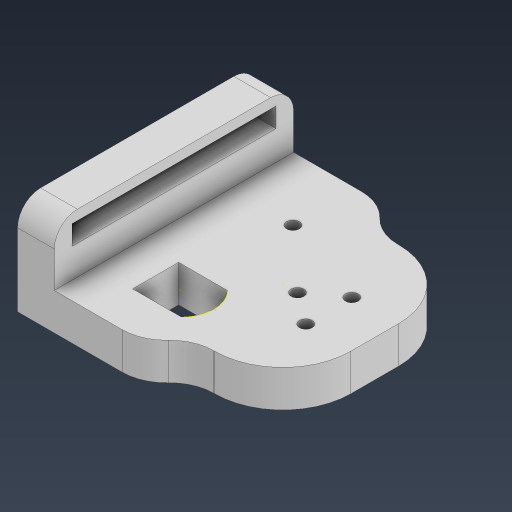
# Autodesk Inventor part: Podstawa
Saved by Autodesk Inventor 2024 (Build 280153000, 153)
## iProperties
Created: 2023-12-19
Part Number: Podstawa
Material: Generic
Document SubType Name: Modeling
Designer: Piter
Density: 1 g/cm^3
Appearance: Default
Author: Piter
Autodesk Inventor part; units mm, degrees
ref_plane "YZ Plane" through (0, 0, 0) normal (1, 0, 0) x (0, 1, 0)
ref_plane "XZ Plane" through (0, 0, 0) normal (0, 1, 0) x (-1, 0, 0)
ref_plane "XY Plane" through (0, 0, 0) normal (0, 0, 1) x (1, 0, 0)
sketch "Sketch1" plane through (0, 0, 0) normal (0, 1, 0) x (-1, 0, 0)
  line L0 (-25, 25) -> (25, 25)
  line L1 (25, 25) -> (25, -25)
  line L2 (25, -25) -> (-25, -25)
  line L3 (-25, -25) -> (-25, 25)
  line L4 (-25, 25) -> (25, -25) construction
  line L5 (25, 25) -> (-25, -25) construction
  line L6 (25, 0) -> (-25, 0)
  circle A0 centre (12.5, 15.25) radius 1.75
  line L7 (-25, 12.5) -> (0, 12.5)
  line L8 (-12.5, 12.5) -> (-12.5, 0)
  circle A1 centre (-12.5, 6.25) radius 1.75
  line L9 (25, -25) -> (-25, 25) construction
  circle A2 centre (12.5, -15.25) radius 1.75
  circle A3 centre (-12.5, -6.25) radius 1.75
  line L10 (0, 32.5) -> (50, 32.5)
  line L11 (50, 32.5) -> (50, -32.5)
  line L12 (50, -32.5) -> (0, -32.5)
  line L13 (0, -32.5) -> (0, 32.5)
  line L14 (0, 32.5) -> (50, -32.5) construction
  line L15 (50, 32.5) -> (0, -32.5) construction
  line L16 (50, -32.5) -> (29.5652, -32.5)
  line L17 (29.5652, -32.5) -> (29.5652, 32.5)
  line L18 (29.5652, 32.5) -> (50, 32.5)
  line L19 (50, 32.5) -> (50, -32.5)
  line L20 (0, 32.5205) -> (0, -32.5)
  circle A4 centre (12.5, -15.25) radius 15
  line L21 (29.5652, -32.5) -> (39.5652, -32.5)
  line L22 (39.5652, -32.5) -> (39.5652, 32.5)
  line L23 (39.5652, 32.5) -> (29.5652, 32.5)
  line L24 (29.5652, 32.5) -> (29.5652, -32.5)
  line L25 (12.5, -15.25) -> (12.5, 0)
  line L26 (-12.5, -6.25) -> (12.5, -6.25)
  circle A5 centre (-4, 0) radius 5
  circle A6 centre (-4, 0) radius 1.75
  line L27 (0, 0) -> (-4, 0)
  point P0 (0, -12.5)
  point P1 (-12.5, -12.5)
  point P2 (0, 25)
  point P3 (0, -25)
  point P4 (0, 25)
  point P5 (0, -25)
  point P6 (0, 32.5)
  point P7 (0, 32.5)
  point P8 (0, -23.5416)
  point P9 (1.101, -25)
  point P10 (25, -23.5416)
  point P11 (23.899, -25)
  point P12 (39.5652, 32.5)
  point P13 (0, 0)
  dimension "d0" = 50
  dimension "d1" = 50
  dimension "d5" = 3.5
  dimension "d7" = 3.5
  dimension "d11" = 15.25
  dimension "d12" = 50
  dimension "d13" = 65
  dimension "d19" = 30
  dimension "d21" = 10
  dimension "d27" = 7.5
  dimension "d28" = 7.5
  dimension "d31" = 9
  dimension "d32" = 25
  dimension "d57" = 10
  dimension "d58" = 3.5
  dimension "d59" = 4
  constraints: 56 end point, 9 midpoint, 9 parallel, 7 centre point, 7 point on line, 6 perpendicular, 4 horizontal, 4 symmetric about line, 2 coincident, 1 vertical, 2 other
  measures "d0" distance of L1.end L2.end
  measures "d1" distance of L0.end L1.end
  measures "d5" diameter of A0
  measures "d7" diameter of A1
  measures "d11" distance from line of A0.centre L6
  measures "d12" distance of L11.end L12.end
  measures "d13" distance of L10.end L11.end
  measures "d19" diameter of A4
  measures "d21" distance of L23.end L22.end
  measures "d27" distance between parallel lines of L2 L12
  measures "d28" distance between parallel lines of L0 L10
  measures "d31" distance from line of L26 A2.centre
  measures "d32" distance of L26.start L26.end
  measures "d57" diameter of A5
  measures "d58" diameter of A6
  measures "d59" distance of point (0, 0) L27.end
extrude "Extrusion3" add sketch "Sketch1" along normal blind 10 contours L0 L13 L7 L3 | L13 L10 L17 L12 L2 A4 L1 L0 | L0 L1 L6 A5 L13 | L7 L8 A1 L6 L3 | L13 A5 L6 L8 A1 L7 | L6 A5 L13 A4 L2 L3 | L1 A4 L25 L6 | A5 L6 L13 | L13 L6 A6 A5 | A4 L1 | L1 A4 L2 L13 L26 L25 | L25 A4 L26 L13 A5 L6 | L13 A5 L6 A6 | L6 A5 L13 | L13 A4 L2 | L1 L2 A4 | L25 L26 A4 | L2 A4 | A4 L13 | A4 L13 L26
extrude "Extrusion4" add sketch "Sketch1" along normal blind 26 contours L10 L22 L12 L17
fillet "Fillet5" radius 12 2 edges at (0, 5, 32.5) (0, 5, -32.5)
fillet "Fillet6" radius 12 2 edges at (0, 5, 25) (0, 5, -25)
fillet "Fillet7" radius 18.5 2 edges at (25, 5, 25) (25, 5, -25)
sketch "Sketch2" plane through (0, 10, 0) normal (0, 1, 0) x (1, 0, 0)
  circle A0 centre (-12.5, -15.25) radius 1.75 projected
  circle A1 centre (-12.5, -15.25) radius 9
  line L0 (-21.5, -15.25) -> (1.5, -15.25)
  line L1 (1.5, -15.25) -> (3.5, -15.25)
  circle A2 centre (3.5, -15.25) radius 1
  line L2 (-21.5, -15.25) -> (-23.5, -15.25)
  circle A3 centre (-23.5, -15.25) radius 1
  point P0 (0, 0)
  dimension "d34" = 18
  dimension "d45" = 23
  dimension "d46" = 2
  dimension "d47" = 2
  dimension "d48" = 2
  dimension "d49" = 2
  constraints: 6 end point, 3 coincident, 3 horizontal, 2 centre point, 1 horizontal alignment, 2 other
  measures "d45" distance of L0.start L0.end
  measures "d46" distance of L0.end L1.end
  measures "d47" diameter of A2
  measures "d48" distance of L0.start L2.end
  measures "d49" diameter of A3
extrude "Extrusion5" cut sketch "Sketch2" against normal blind 7 contours L0 A1 A0 | A0 L0 A1
sketch "Sketch3" plane through (-29.5652, 10, -32.5) normal (1, 0, 0) x (0, 0, -1)
  line L0 (0, 0) -> (-65, 0) projected
  line L1 (-65, 0) -> (-65, 8)
  line L2 (-65, -10) -> (-65, 16) projected
  line L3 (-65, 8) -> (0, 8)
  line L4 (-65, 8) -> (-60.2, 8)
  line L5 (-60.2, 8) -> (-4.8, 8)
  line L6 (-4.8, 8) -> (-4.8, 13.3)
  line L7 (-4.8, 13.3) -> (-60.2, 13.3)
  line L8 (-60.2, 13.3) -> (-60.2, 8)
  point P0 (-32.5, -10)
  point P1 (-4.8, 8)
  dimension "d37" = 8
  dimension "d38" = 65
  dimension "d39" = 4.8
  dimension "d40" = 55.4
  dimension "d41" = 5.3
  constraints: 14 end point, 2 parallel, 2 perpendicular, 2 point on line, 1 horizontal
  measures "d37" distance of L0.end L1.end
  measures "d38" distance of L1.end L3.end
  measures "d39" distance of L1.end L4.end
  measures "d40" distance of L7.end L6.end
  measures "d41" distance of L6.end L5.end
extrude "Extrusion6" cut sketch "Sketch3" against normal through all
fillet "Fillet8" radius 6.25 2 edges at (-34.5652, 26, 32.5) (-34.5652, 26, -32.5)
sketch "Sketch4" plane through (-12.5, 3, 15.25) normal (0, 1, 0) x (1, 0, 0)
  circle A0 centre (0, 0) radius 9 projected
  line L0 (-7.65, -7.5) -> (14.85, -7.5)
  line L1 (14.85, -7.5) -> (14.85, 7.5)
  line L2 (0, 0) -> (-6.8, 0)
  line L3 (-6.8, 0) -> (-6.8, 6.25)
  line L4 (-6.8, 6.25) -> (16.5, 6.25)
  line L5 (16.5, 6.25) -> (16.5, -6.25)
  line L6 (16.5, -6.25) -> (-6.8, -6.25)
  line L7 (-6.8, -6.25) -> (-6.8, 6.25)
  point P0 (12.5, 15.25)
  point P1 (-9, 0)
  point P2 (-6.8, 0)
  point P3 (14.85, -6.25)
  point P4 (14.85, 6.25)
  dimension "d50" = 22.5
  dimension "d51" = 15
  dimension "d66" = 6.8
  dimension "d67" = 6.25
  dimension "d68" = 23.3
  dimension "d69" = 12.5
  constraints: 16 end point, 2 horizontal, 2 parallel, 2 perpendicular, 1 horizontal alignment, 1 vertical, 1 other
  measures "d50" distance of L0.start L0.end
  measures "d51" distance of L0.end L1.end
  measures "d66" distance of L2.start L2.end
  measures "d67" distance of L2.end L3.end
  measures "d68" distance of L5.end L6.end
  measures "d69" distance of L4.end L5.end
sketch "Sketch5" plane through (-39.5652, 0, 32.5) normal (0, -1, 0) x (1, 0, 0)
  circle A0 centre (52.0652, -26.25) radius 1.75 projected
  circle A1 centre (52.0652, -26.25) radius 3.5
  circle A2 centre (52.0652, -38.75) radius 1.75 projected
  circle A3 centre (52.0652, -38.75) radius 3.5
  circle A4 centre (43.5652, -32.5) radius 1.75 projected
  circle A5 centre (43.5652, -32.5) radius 3.5
  circle A6 centre (27.0652, -47.75) radius 1.75 projected
  circle A7 centre (27.0652, -47.75) radius 3.5
  point P0 (39.5652, -32.5)
  dimension "d60" = 7
  dimension "d61" = 7
  dimension "d62" = 7
  dimension "d63" = 7
  constraints: 4 centre point, 4 coincident
  measures "d60" diameter of A1
  measures "d61" diameter of A3
  measures "d62" diameter of A5
  measures "d63" diameter of A7
extrude "Extrusion8" cut sketch "Sketch5" against normal blind 5 contours A1 | A3 | A4 | A5 | A7
extrude "Extrusion9" cut sketch "Sketch4" against normal through all contours A0 L6 L7 L3 L4 | A0 L4 L1 L6 | A0 L3 L4 | L4 L5 L6 L1 | L6 L7 A0
move faces "Move2" translate (0, 7, 0) faces at (-14.1282, 3, 8.5636) (-20.0333, 3, 15.25) (-14.1282, 3, 21.9364)
sketch "Sketch7" plane through (-29.5652, 10, -32.5) normal (0, 1, 0) x (1, 0, 0)
  arc A0 (23.5411, -54) -> (23.5411, -41.5) centre (17.0652, -47.75) ccw projected
  point P0 (29.5652, -32.5)
  point P1 (26.0652, -47.75)
  constraints: 1 point on circle
move faces "Move3" translate (0, 9.5, 0) faces at (-19.1934, 3, 21.3832)
move faces "Move4" translate (0, 12.5, 0) faces at (-19.1934, 3, 9.1168)
body "Solid2"
